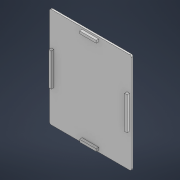
# Autodesk Inventor part: LightCasingLid
Saved by Autodesk Inventor 2021 (Build 250183000, 183)
## iProperties
Created: 2022-01-15
Part Number: LightCasingLid
Material: Generic
Document SubType Name: Sheet Metal
Designer: ivanl
Density: 1 g/cm^3
Sheet Metal Rule: Default
Appearance: Default
Author: ivanl
## iProperties of the stored document _3DPrint.ipt
Created: 2022-01-15
Part Number: _3DPrint
Material: Generic
Document SubType Name: Modeling
Designer: ivanl
Density: 1 g/cm^3
Appearance: Default
Author: ivanl
Autodesk Inventor part; units mm, degrees
ref_plane "YZ Plane" through (0, 0, 0) normal (1, 0, 0) x (0, 1, 0)
ref_plane "XZ Plane" through (0, 0, 0) normal (0, 1, 0) x (-1, 0, 0)
ref_plane "XY Plane" through (0, 0, 0) normal (0, 0, 1) x (1, 0, 0)
sketch "Sketch1" plane through (0, 0, 0) normal (0, 0, 1) x (1, 0, 0)
  line L0 (-49.5, 60.5) -> (49.5, 60.5)
  line L1 (49.5, 60.5) -> (49.5, -60.5)
  line L2 (49.5, -60.5) -> (-49.5, -60.5)
  line L3 (-49.5, -60.5) -> (-49.5, 60.5)
  line L4 (-49.5, 60.5) -> (49.5, -60.5) construction
  line L5 (49.5, 60.5) -> (-49.5, -60.5) construction
  point P0 (0, 0)
  dimension "d0" = 99
  dimension "d1" = 121
  constraints: 12 end point, 2 midpoint, 2 parallel, 1 horizontal, 1 perpendicular
  measures "d0" distance of L0.start L0.end
  measures "d1" distance of L0.end L1.end
extrude "Extrusion1" add sketch "Sketch1" along normal blind 2
sketch "Sketch2" plane through (0, 0, 2) normal (0, 0, 1) x (1, 0, 0)
  line L0 (-47.3, 58.3) -> (47.3, 58.3)
  line L1 (47.3, 58.3) -> (47.3, -58.3)
  line L2 (47.3, -58.3) -> (-47.3, -58.3)
  line L3 (-47.3, -58.3) -> (-47.3, 58.3)
  line L4 (-47.3, 58.3) -> (47.3, -58.3) construction
  line L5 (47.3, 58.3) -> (-47.3, -58.3) construction
  point P0 (0, 0)
  dimension "d4" = 116.6
  dimension "d5" = 94.6
  constraints: 12 end point, 2 midpoint, 2 parallel, 1 horizontal, 1 perpendicular
  measures "d4" distance of L0.end L1.end
  measures "d5" distance of L0.start L0.end
extrude "Extrusion2" add sketch "Sketch2" along normal blind 3
fillet "Fillet1" radius 2 4 edges at (49.5, 60.5, 1) (-49.5, 60.5, 1) (49.5, -60.5, 1) (-49.5, -60.5, 1)
sketch "Sketch5" plane through (0, 0, 5) normal (0, 0, 1) x (1, 0, 0)
  line L0 (44.3, -55.3) -> (-44.3, -55.3)
  line L1 (-44.3, -55.3) -> (-44.3, 55.3)
  line L2 (-44.3, 55.3) -> (44.3, 55.3)
  line L3 (44.3, 55.3) -> (44.3, -55.3)
  line L4 (44.3, -55.3) -> (-44.3, 55.3) construction
  line L5 (-44.3, -55.3) -> (44.3, 55.3) construction
  line L6 (47.3, 58.3) -> (-47.3, 58.3) projected
  line L7 (47.3, -58.3) -> (47.3, 58.3) projected
  line L8 (-78.6, 90.6) -> (-10, 90.6)
  line L9 (-10, 90.6) -> (-10, 20)
  line L10 (-10, 20) -> (-78.6, 20)
  line L11 (-78.6, 20) -> (-78.6, 90.6)
  line L12 (-78.6, 90.6) -> (-10, 20) construction
  line L13 (-10, 90.6) -> (-78.6, 20) construction
  line L14 (78.6, 90.6) -> (10, 90.6)
  line L15 (10, 90.6) -> (10, 20)
  line L16 (10, 20) -> (78.6, 20)
  line L17 (78.6, 20) -> (78.6, 90.6)
  line L18 (78.6, 90.6) -> (10, 20) construction
  line L19 (10, 90.6) -> (78.6, 20) construction
  line L20 (10, -20) -> (78.6, -20)
  line L21 (78.6, -20) -> (78.6, -90.6)
  line L22 (78.6, -90.6) -> (10, -90.6)
  line L23 (10, -90.6) -> (10, -20)
  line L24 (10, -20) -> (78.6, -90.6) construction
  line L25 (78.6, -20) -> (10, -90.6) construction
  line L26 (-78.6, -90.6) -> (-10, -90.6)
  line L27 (-10, -90.6) -> (-10, -20)
  line L28 (-10, -20) -> (-78.6, -20)
  line L29 (-78.6, -20) -> (-78.6, -90.6)
  line L30 (-78.6, -90.6) -> (-10, -20) construction
  line L31 (-10, -90.6) -> (-78.6, -20) construction
  point P0 (0, 0)
  point P1 (-10, -55.3)
  point P2 (-44.3, -20)
  point P3 (44.3, -20)
  point P4 (10, -55.3)
  point P5 (-44.3, 20)
  point P6 (-10, 55.3)
  point P7 (10, 55.3)
  point P8 (44.3, 20)
  dimension "d23" = 3
  dimension "d24" = 3
  dimension "d27" = 20
  dimension "d28" = 40
  constraints: 60 end point, 10 midpoint, 10 parallel, 6 collinear, 5 horizontal, 5 perpendicular
  measures "d23" distance between parallel lines of L6 L2
  measures "d24" distance between parallel lines of L7 L3
  measures "d27" distance between parallel lines of L15 L9
  measures "d28" distance between parallel lines of L16 L20
extrude "Extrusion5" cut sketch "Sketch5" against normal up to surface (3 mm away) contours L3 L20 L21 L22 L23 L0 | L0 L23 L20 L3 | L0 L27 L28 L1 L10 L9 L2 L15 L16 L3 L20 L23 | L27 L26 L29 L28 L1 L0 | L0 L1 L28 L27 | L16 L15 L2 L3 | L3 L2 L15 L6 L7 L16 | L7 L6 L15 L14 L17 L16 | L10 L11 L8 L9 L2 L1 | L1 L2 L9 L10
equation "\"BendRadius\" = Thickness"
equation "\"BendReliefWidth\" = Thickness"
equation "\"BendReliefDepth\" = 0.5 * Thickness"
equation "\"CornerReliefSize\" = 4 * Thickness"
equation "\"MinimumRemnant\" = 2 * Thickness"
equation "\"TransitionRadius\" = BendRadius"
equation "\"JacobiRadiusSize\" = BendRadius"
equation "\"GapSize\" = Thickness"
equation "\"Thickness\" = 3.048"
body "Solid1"
